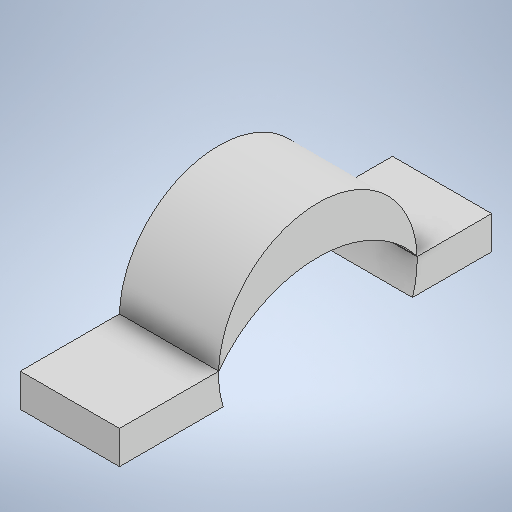
# Autodesk Inventor part: secures
Saved by Autodesk Inventor 2025.3 (Build 293356030, 356C)
## iProperties
Created: 2026-06-24
Part Number: secures
Material: Generic
Document SubType Name: Modeling
Designer: user
Density: 1 g/cm^3
Appearance: Default
Author: user
Autodesk Inventor part; units mm, degrees
ref_plane "YZ Plane" through (0, 0, 0) normal (1, 0, 0) x (0, 1, 0)
ref_plane "XZ Plane" through (0, 0, 0) normal (0, 1, 0) x (-1, 0, 0)
ref_plane "XY Plane" through (0, 0, 0) normal (0, 0, 1) x (1, 0, 0)
sketch "Sketch1" plane through (0, 0, 0) normal (1, 0, 0) x (0, 1, 0)
  line L0 (0, 0) -> (10, 0)
  line L1 (10, 0) -> (10, -30)
  line L2 (0, 0) -> (0, -20)
  arc A0 (0, -88.586) -> (0, -31.3842) centre (9.0549, -59.9851) ccw
  line L3 (10, -82.5554) -> (10, -112.5554)
  line L4 (10, -112.5554) -> (0, -112.5554)
  line L5 (0, -112.5554) -> (0, -88.586)
  line L6 (0, -31.3842) -> (0, -20)
  arc A1 (10.1476, -89.9652) -> (10, -30) centre (-13.0468, -60.0395) ccw
  point P0 (10, -26.568)
  point P1 (10, -89.9702)
  dimension "d0" = 10
  dimension "d1" = 30
  dimension "d2" = 20
  dimension "d3" = 30
  dimension "d6" = 30
  dimension "d7" = 10
  constraints: 14 end point, 6 point on circle, 2 centre point, 2 perpendicular, 1 collinear, 1 horizontal, 1 point on line, 1 vertical
  measures "d0" distance of L0.start L0.end
  measures "d1" distance of L0.end L1.end
  measures "d2" distance of L0.start L2.end
  measures "d3" distance of L3.start L3.end
  measures "d6" radius of A0
  measures "d7" distance of L3.end L4.end
extrude "Extrusion1" add sketch "Sketch1" along normal blind 30 contours L3 L4 L5 A0 | L0 L1 A0 L6 L2
extrude "Extrusion2" add sketch "Sketch1" along normal blind 30 contours A0 A1
body "Solid1"
